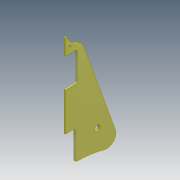
# Autodesk Inventor part: tampa frontal - corpo
Saved by Autodesk Inventor 2016 (Build 200138000, 138)
## iProperties
Created: 2018-12-06
Part Number: tampa frontal - corpo
Material: Generic
Document SubType Name: Modeling
Designer: lesly
Density: 1 g/cm^3
Appearance: Yellow(1)
Author: lesly
Autodesk Inventor part; units mm, degrees
ref_plane "YZ Plane" through (0, 0, 0) normal (1, 0, 0) x (0, 1, 0)
ref_plane "XZ Plane" through (0, 0, 0) normal (0, 1, 0) x (-1, 0, 0)
ref_plane "XY Plane" through (0, 0, 0) normal (0, 0, 1) x (1, 0, 0)
ref_plane "Work Plane3" through (-50, 0, 0) normal (-1, 0, 0) x (0, 0, 1)
sketch "Sketch6" plane through (-50, 0, 0) normal (-1, 0, 0) x (0, 0, 1)
  arc A0 (-92.5702, 77.4165) -> (-109.8479, 59.8803) centre (-96.1815, 63.695) ccw
  line L0 (-70.536, 69.486) -> (-92.5702, 77.4165)
  line L1 (44.1213, 28.2183) -> (-70.536, 69.486)
  arc A1 (53.2724, 20) -> (44.1213, 28.2183) centre (36.052, 10.0292) ccw
  arc A2 (53.2724, 20) -> (69.1541, 1.9881) centre (80.7478, 28.2183) ccw
  arc A3 (69, 0) -> (69.1541, 1.9881) centre (69, 1) ccw
  line L2 (45, 0) -> (69, 0)
  line L3 (45, 15) -> (45, 0)
  arc A4 (45, 15) -> (42, 18) centre (42, 15) ccw
  line L4 (3, 18) -> (42, 18)
  arc A5 (3, 18) -> (0, 15) centre (3, 15) ccw
  line L5 (0, 0) -> (0, 15)
  line L6 (0, 0) -> (-59.2, 0)
  line L7 (-59.2, 0) -> (-59.2, 12)
  arc A6 (-59.2, 12) -> (-62.2, 15) centre (-62.2, 12) ccw
  line L8 (-62.2, 15) -> (-101.1648, 15)
  arc A7 (-104.1648, 18.006) -> (-101.1648, 15) centre (-101.1648, 18) ccw
  arc A8 (-104.1648, 18.006) -> (-109.8479, 59.8803) centre (-258.9764, 18.3179) ccw
  constraints: 18 end point, 18 point on circle, 9 centre point
extrude "Extrusion2" add sketch "Sketch6" along normal blind 2
sketch "Sketch7" plane through (-50, 0, 0) normal (1, 0, 0) x (0, 0, -1)
  circle A0 centre (75.7329, 49.2486) radius 2.5
  circle A1 centre (-53.2724, 6.5547) radius 1.5
  point P0 (0, 0)
  constraints: 2 centre point, 2 coincident
extrude "Extrusion3" cut sketch "Sketch7" against normal blind 10
chamfer "Chamfer1" distance 2 angle 45 1 edges at (-50, 49.2486, -73.2329)
chamfer "Chamfer2" distance 1 angle 45 1 edges at (-50, 6.5547, 54.7724)
body "Solid1"
